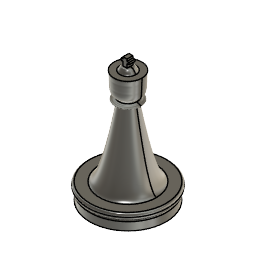
Rege (Autodesk Fusion 360 design; units mm, degrees)
part number: 2026-03-27-19-00-09-599
Autodesk Fusion 360 part; units mm, degrees
sketch "Rege" plane through (0, 0, 0) normal (0, 1, 0) x (1, 0, 0)
  line L0 (0, 0) -> (19, 0)
  line L1 (0, 0) -> (0, -60)
  line L2 (0, 0) -> (19, 0)
  line L3 (19, 0) -> (19, -4)
  line L4 (18, -5) -> (0, -5)
  line L5 (0, -5) -> (0, 0)
  line L6 (0, -5) -> (19, -5)
  line L7 (18.9974, -7.9995) -> (0, -7.9995)
  line L8 (0, -7.9995) -> (0, -5)
  arc A0 (18.9974, -7.9995) -> (19.8649, -6.502) centre (18.9974, -6.9995) ccw
  arc A1 (19.8649, -6.502) -> (19, -5) centre (19, -6) ccw
  arc A2 (18, -5) -> (19, -4) centre (18, -4) ccw
  line L9 (0, -60) -> (0, -48)
  line L10 (0, -60) -> (0, -40)
  line L11 (0, -37.8406) -> (0, -40)
  line L12 (0, -40) -> (0, -43.0218)
  line L13 (0, -44.611) -> (4.5124, -44.611)
  line L14 (0, -43.0218) -> (0, -44.611)
  spline S0 degree 5 poles (4.3, -42.4) (4.5854, -40.7333) (5.1533, -37.4872) (5.9962, -32.8797) (7.1016, -27.2682) (8.4509, -21.2027) (9.7649, -16.1777) (11.041, -12.29) (12.2781, -9.611) (13.4785, -8.1257) (14.6503, -7.6865) (15.5797, -7.8283) (16.2833, -7.9459) (16.757, -7.9878) (16.995, -7.9995) knots 0 0 0 0 0 0 0.1 0.2 0.3 0.4 0.5 0.6 0.7 0.8 0.9 1 1 1 1 1 1
  line L15 (13.1828, -7.8119) -> (20.8072, -8.1871)
  line L16 (0, -62) -> (1, -62)
  line L17 (1, -62) -> (1, -61)
  line L18 (1, -61) -> (2, -61)
  line L19 (2, -61) -> (2, -60)
  line L20 (2, -60) -> (1, -60)
  line L21 (1, -60) -> (1, -58)
  line L22 (1, -58) -> (0, -58)
  line L23 (0, -60) -> (0, -62)
  spline S1 degree 5 poles (1, -58) (1.0261, -58.002) (1.0784, -58.0057) (1.157, -58.0102) (1.2626, -58.0139) (1.3953, -58.0148) (1.5285, -58.0119) (1.6613, -58.0054) (1.7923, -57.9951) (1.9194, -57.9812) (2.0399, -57.9637) (2.1511, -57.9425) (2.2509, -57.9175) (2.3386, -57.8882) (2.4148, -57.8537) (2.4825, -57.8127) (2.5449, -57.7643) (2.6056, -57.7078) (2.6673, -57.6437) (2.731, -57.5736) (2.7967, -57.4997) (2.8633, -57.4243) (2.9296, -57.3492) (2.9944, -57.2749) (3.0568, -57.2001) (3.1167, -57.1232) (3.174, -57.0419) (3.2294, -56.9548) (3.284, -56.8615) (3.3394, -56.7629) (3.3975, -56.6609) (3.4601, -56.5577) (3.529, -56.4553) (3.6054, -56.3556) (3.6901, -56.2596) (3.7837, -56.1679) (3.8657, -56.0984) (3.9313, -56.0483) (3.9768, -56.016) (4, -56) knots 0 0 0 0 0 0 0.028571 0.057143 0.085714 0.114286 0.142857 0.171429 0.2 0.228571 0.257143 0.285714 0.314286 0.342857 0.371429 0.4 0.428571 0.457143 0.485714 0.514286 0.542857 0.571429 0.6 0.628571 0.657143 0.685714 0.714286 0.742857 0.771429 0.8 0.828571 0.857143 0.885714 0.914286 0.942857 0.971429 1 1 1 1 1 1
  line L24 (4, -56) -> (7, -56)
  spline S2 degree 5 poles (4.5124, -44.611) (4.5363, -44.6464) (4.5836, -44.7159) (4.6528, -44.8164) (4.7418, -44.9431) (4.8473, -45.0892) (4.9477, -45.2239) (5.0436, -45.3482) (5.1363, -45.4642) (5.2275, -45.575) (5.3196, -45.6843) (5.4142, -45.7953) (5.5127, -45.9104) (5.6149, -46.0299) (5.7192, -46.1519) (5.823, -46.2737) (5.9236, -46.3925) (6.0183, -46.5068) (6.1055, -46.6173) (6.1842, -46.7269) (6.2544, -46.8393) (6.3163, -46.9576) (6.3707, -47.0832) (6.4186, -47.2156) (6.461, -47.3527) (6.499, -47.4924) (6.5334, -47.6329) (6.5651, -47.7744) (6.5944, -47.9176) (6.6216, -48.0643) (6.6465, -48.216) (6.6688, -48.3742) (6.6877, -48.5393) (6.7026, -48.7114) (6.7132, -48.8904) (6.7193, -49.0755) (6.722, -49.266) (6.7227, -49.4608) (6.7233, -49.6587) (6.7255, -49.8585) (6.7307, -50.0587) (6.7396, -50.2577) (6.7516, -50.4538) (6.7655, -50.6453) (6.7796, -50.831) (6.7923, -51.0103) (6.8026, -51.1836) (6.8102, -51.3526) (6.8158, -51.5199) (6.8207, -51.6886) (6.8259, -51.8614) (6.8323, -52.0401) (6.8399, -52.2248) (6.8478, -52.4137) (6.8548, -52.6045) (6.8598, -52.7945) (6.8622, -52.9814) (6.8623, -53.1645) (6.8615, -53.3447) (6.862, -53.5237) (6.866, -53.704) (6.8752, -53.8879) (6.8906, -54.0768) (6.9114, -54.2708) (6.9362, -54.469) (6.9623, -54.6696) (6.9871, -54.8706) (7.008, -55.0699) (7.0229, -55.266) (7.0304, -55.4576) (7.0296, -55.6442) (7.0222, -55.7893) (7.0126, -55.8956) (7.0045, -55.9654) (7, -56) knots 0 0 0 0 0 0 0.01428571 0.02857143 0.04285714 0.05714286 0.07142857 0.08571429 0.1 0.11428571 0.12857143 0.14285714 0.15714286 0.17142857 0.18571429 0.2 0.21428571 0.22857143 0.24285714 0.25714286 0.27142857 0.28571429 0.3 0.31428571 0.32857143 0.34285714 0.35714286 0.37142857 0.38571429 0.4 0.41428571 0.42857143 0.44285714 0.45714286 0.47142857 0.48571429 0.5 0.51428571 0.52857143 0.54285714 0.55714286 0.57142857 0.58571429 0.6 0.61428571 0.62857143 0.64285714 0.65714286 0.67142857 0.68571429 0.7 0.71428571 0.72857143 0.74285714 0.75714286 0.77142857 0.78571429 0.8 0.81428571 0.82857143 0.84285714 0.85714286 0.87142857 0.88571429 0.9 0.91428571 0.92857143 0.94285714 0.95714286 0.97142857 0.98571429 1 1 1 1 1 1
  line L25 (11, -41.5218) -> (11, -41.5)
  line L26 (0, -42.4) -> (4.7, -42.4)
  line L27 (0, -44.611) -> (4.5124, -44.611)
  spline S3 degree 5 poles (4.5124, -44.611) (4.5154, -44.5998) (4.5227, -44.5779) (4.5373, -44.5462) (4.5641, -44.5064) (4.6099, -44.4604) (4.6672, -44.4181) (4.7346, -44.3788) (4.8099, -44.3414) (4.8897, -44.3046) (4.971, -44.2668) (5.0508, -44.2273) (5.1275, -44.1854) (5.2013, -44.1421) (5.274, -44.0992) (5.3486, -44.0588) (5.428, -44.0231) (5.514, -43.9937) (5.6068, -43.9707) (5.7039, -43.9528) (5.8016, -43.9376) (5.8956, -43.9226) (5.9825, -43.9055) (6.0599, -43.8852) (6.1285, -43.8623) (6.1907, -43.8388) (6.2497, -43.8166) (6.3077, -43.7971) (6.3652, -43.7795) (6.4194, -43.7609) (6.4664, -43.7371) (6.502, -43.7046) (6.5232, -43.6622) (6.5297, -43.6119) (6.523, -43.5581) (6.5052, -43.5053) (6.4782, -43.4569) (6.4424, -43.4129) (6.397, -43.3711) (6.3413, -43.3284) (6.2746, -43.2819) (6.1975, -43.2306) (6.1117, -43.1754) (6.0196, -43.1187) (5.924, -43.0634) (5.8277, -43.0123) (5.7327, -42.9673) (5.64, -42.9285) (5.5496, -42.8945) (5.4611, -42.8628) (5.3731, -42.8306) (5.2847, -42.7948) (5.1946, -42.7526) (5.1021, -42.7024) (5.0067, -42.6428) (4.9081, -42.5731) (4.8266, -42.5091) (4.7639, -42.4564) (4.7214, -42.4191) (4.7, -42.4) knots 0 0 0 0 0 0 0.018182 0.036364 0.054545 0.072727 0.090909 0.109091 0.127273 0.145455 0.163636 0.181818 0.2 0.218182 0.236364 0.254545 0.272727 0.290909 0.309091 0.327273 0.345455 0.363636 0.381818 0.4 0.418182 0.436364 0.454545 0.472727 0.490909 0.509091 0.527273 0.545455 0.563636 0.581818 0.6 0.618182 0.636364 0.654545 0.672727 0.690909 0.709091 0.727273 0.745455 0.763636 0.781818 0.8 0.818182 0.836364 0.854545 0.872727 0.890909 0.909091 0.927273 0.945455 0.963636 0.981818 1 1 1 1 1 1
  line L28 (0, -62) -> (-1, -62)
  line L29 (-1, -62) -> (-1, -61)
  line L30 (-1, -61) -> (-2, -61)
  line L31 (-2, -61) -> (-2, -60)
  line L32 (-2, -60) -> (-1, -60)
  line L33 (-1, -60) -> (-1, -58)
  line L34 (-1, -58) -> (0, -58)
  point P0 (14.0855, -7.9995)
  point P1 (1.7236, -58)
  point P2 (2.3, -57.9)
  point P3 (2.6058, -57.706)
  point P4 (2.91, -57.3713)
  point P5 (3.2, -57)
  point P6 (3.5, -56.5)
  point P7 (5.0617, -45.3702)
  point P8 (5.4826, -45.8753)
  point P9 (5.9597, -46.4365)
  point P10 (6.2959, -46.9218)
  point P11 (6.5, -47.5)
  point P12 (6.6352, -48.1496)
  point P13 (6.716, -48.9897)
  point P14 (6.7321, -50.0721)
  point P15 (6.7967, -51.0899)
  point P16 (6.8291, -51.9461)
  point P17 (6.8614, -52.9478)
  point P18 (6.8775, -53.9009)
  point P19 (7, -55)
  point P20 (4.7, -44.4)
  point P21 (5.1, -44.2)
  point P22 (5.5, -44)
  point P23 (6, -43.9)
  point P24 (6.3, -43.8)
  point P25 (6.5, -43.7)
  point P26 (6.5, -43.5)
  point P27 (6.3, -43.3)
  point P28 (5.8, -43)
  point P29 (5.3, -42.8)
  dimension "d1" = 19
  dimension "d2" = 1
  dimension "d3" = 20
  dimension "d5" = 2
  constraint coincident L0.start L1.start
  constraint horizontal L0
  constraint perpendicular L0 L1
  constraint horizontal L2
  constraint vertical L3
  constraint horizontal L4
  constraint vertical L5
  constraint horizontal L6
  constraint horizontal L7
  constraint vertical L8
  constraint tangent L7 A0
  constraint tangent L6 A1
  constraint equal A0 A1
  constraint coincident A0.end A1.start
  constraint tangent L3 A2
  constraint tangent L4 A2
  constraint equal A0 A2
  constraint coincident L1 L9.end
  constraint parallel L1 L10
  constraint vertical L11
  constraint vertical L12
  constraint coincident L1 L12.end
  constraint horizontal L13
  constraint vertical L14
  constraint coincident L1 L13.start
  constraint coincident L7 S0.end
  constraint midpoint S0.end L15
  constraint perpendicular L10 L16
  constraint perpendicular L16 L17
  constraint perpendicular L17 L18
  constraint perpendicular L18 L19
  constraint perpendicular L17 L20
  constraint perpendicular L20 L21
  constraint coincident L10 L22.end
  constraint perpendicular L16 L23
  constraint perpendicular L9 L24
  constraint coincident L7 P0
  constraint coincident L1 L26.start
  constraint perpendicular L12 L26
  constraint perpendicular L1 L27
  constraint coincident S0.start L26
  constraint perpendicular L23 L28
  constraint perpendicular L28 L29
  constraint perpendicular L29 L30
  constraint perpendicular L30 L31
  constraint perpendicular L31 L32
  constraint perpendicular L32 L33
  constraint perpendicular L10 L34
  measures "d1" distance of L0.start L0.end
  measures "d2" radius of A0
  measures "d3" distance of L1.end L10.end
  measures "d5" distance of L20.end L21.end
revolve "Revolve1" add sketch "Rege" angle 360 about axis through (0, 0, 0) along (0, 0, 1) contours L0 L1 L2 L3 L4 L5 L6 A2 | L1 L4 L6 L7 L8 A0 A1 S0 | L1 L7 L10 L11 L12 S0 L26 | L7 S0 L15 | S0 L15 | L1 L10 L12 L13 L14 L26 L27 S3 | L1 L9 L10 L13 L22 S1 L24 S2 L27
extrude "Extrude1" add sketch "Rege" along normal blind 1.5 and the other way blind 1.5 contours L1 L9 L10 L16 L17 L18 L19 L20 L21 L22 L23 | L1 L9 L10 L23 L28 L29 L30 L31 L32 L33 L34
named bodies: "Rege"
